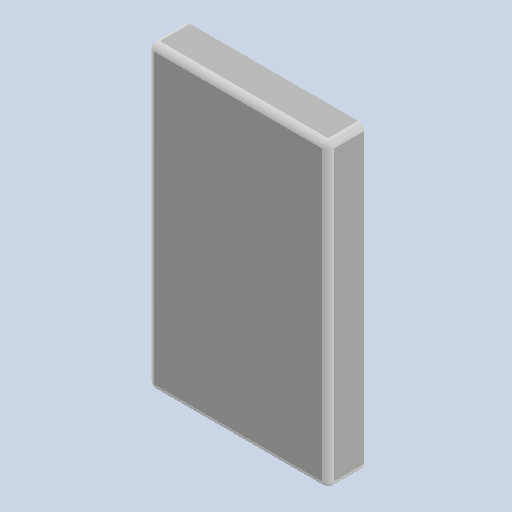
# Autodesk Inventor part: Telit
Saved by Autodesk Inventor 2022 (Build 260153000, 153)
## iProperties
Created: 2022-03-19
Part Number: Telit
Material: Generic
Document SubType Name: Modeling
Designer: dvorakj
Density: 1 g/cm^3
Appearance: Default
Author: dvorakj
Autodesk Inventor part; units mm, degrees
ref_plane "YZ Plane" through (0, 0, 0) normal (1, 0, 0) x (0, 1, 0)
ref_plane "XZ Plane" through (0, 0, 0) normal (0, 1, 0) x (-1, 0, 0)
ref_plane "XY Plane" through (0, 0, 0) normal (0, 0, 1) x (1, 0, 0)
sketch "Sketch1" plane through (0, 0, 0) normal (0, 0, 1) x (1, 0, 0)
  line L0 (7.5, -11.5) -> (-7.5, -11.5)
  line L1 (-7.5, -11.5) -> (-7.5, 13.5)
  line L2 (-7.5, 13.5) -> (7.5, 13.5)
  line L3 (7.5, 13.5) -> (7.5, -11.5)
  line L4 (12.5, 21.5) -> (-9.5, 21.5) projected
  point P0 (0, 0)
  point P1 (0, 13.5)
  dimension "d0" = 15
  dimension "d1" = 25
  dimension "d2" = 8
  constraints: 8 end point, 2 parallel, 1 horizontal, 1 midpoint, 1 perpendicular, 1 vertical alignment
  measures "d0" distance of L1.end L2.end
  measures "d1" distance between parallel lines of L0 L2
  measures "d2" distance between parallel lines of L4 L2
extrude "Extrusion1" add sketch "Sketch1" along normal blind 3
fillet "Fillet1" radius 0.5 4 edges at (0, 13.5, 3) (-7.5, 1, 3) (0, -11.5, 3) (7.5, 1, 3)
fillet "Fillet2" radius 0.5 8 edges at (-7.3536, 13.3536, 2.8536) (-7.5, 13.5, 1.25) (7.3536, 13.3536, 2.8536) (7.5, 13.5, 1.25) (-7.3536, -11.3536, 2.8536) (-7.5, -11.5, 1.25) (7.3536, -11.3536, 2.8536) (7.5, -11.5, 1.25)
body "Solid1"
